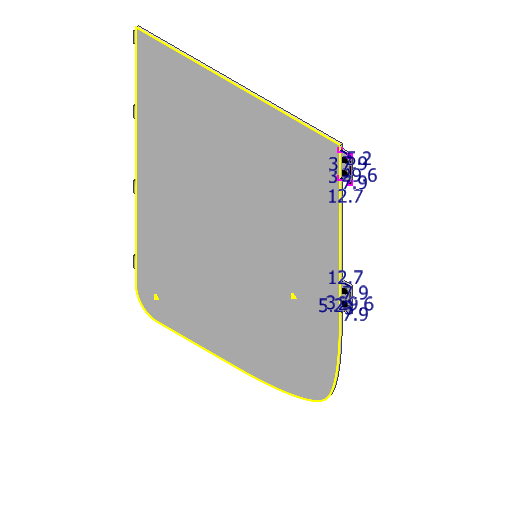
# Autodesk Inventor part: plate cover 1
Saved by Autodesk Inventor 2025.3 (Build 293356030, 356C)
## iProperties
Created: 2025-10-11
Part Number: plate cover 1
Material: 일반
Document SubType Name: Modeling
Designer: joseph
Density: 1 g/cm^3
Appearance: 기본값
Author: joseph
Autodesk Inventor part; units mm, degrees
ref_plane "YZ Plane" through (0, 0, 0) normal (1, 0, 0) x (0, 1, 0)
ref_plane "XZ Plane" through (0, 0, 0) normal (0, 1, 0) x (-1, 0, 0)
ref_plane "XY Plane" through (0, 0, 0) normal (0, 0, 1) x (1, 0, 0)
sketch "스케치1" plane through (0, 0, 0) normal (0, 0, 1) x (1, 0, 0)
  line L0 (-169.6707, -111.8499) -> (-86.0054, -111.8499)
  line L1 (56.3293, 190.1501) -> (-195.6707, 190.1501)
  line L2 (-195.6707, 190.1501) -> (-195.6707, -85.8499)
  arc A0 (-195.6707, -85.8499) -> (-169.6707, -111.8499) centre (-169.6707, -85.8499) ccw
  spline S0 degree 4 poles (76.3293, 10.1501) (76.3293, -29.0333) (69.7342, -103.4516) (54.303, -121.2052) (-24.0976, -131.8499) (-69.6707, -131.8499) knots -3 -3 -3 -3 -3 -2 -1 -1 -1 -1 -1
  line L3 (-169.6707, -111.8499) -> (-69.6707, -111.8499)
  line L4 (56.3293, 10.1501) -> (56.3293, 190.1501)
  line L5 (56.3293, 190.1501) -> (-195.6707, 190.1501)
  line L6 (-195.6707, 190.1501) -> (-195.6707, -85.8499)
  arc A1 (-195.6707, -85.8499) -> (-169.6707, -111.8499) centre (-169.6707, -85.8499) ccw
  spline S1 degree 5 poles (-69.6707, -111.8499) (-63.0133, -111.8499) (-56.3558, -111.7392) (-49.7008, -111.5181) (-37.3206, -110.8938) (-24.9713, -109.8245) (-19.2653, -109.2246) (-9.0381, -107.9323) (1.1128, -106.1432) (5.592, -105.2331) (13.2368, -103.427) (20.711, -101.0169) (23.7891, -99.8797) (28.8563, -97.6943) (33.564, -94.8357) (35.3879, -93.5515) (38.7394, -90.6828) (41.4796, -87.2264) (42.6651, -85.3968) (45.2382, -80.7487) (47.1463, -75.7797) (48.1134, -72.7952) (50.1128, -65.6301) (51.5537, -58.3306) (52.2613, -54.0887) (53.6092, -44.6153) (54.5463, -35.0917) (54.9693, -29.8398) (55.6982, -18.6976) (56.1131, -7.5392) (56.257, -1.6436) (56.3293, 4.2533) (56.3293, 10.1501) knots 0 0 0 0 0 0 0.153999 0.153999 0.153999 0.286688 0.286688 0.286688 0.392369 0.392369 0.392369 0.46822 0.46822 0.46822 0.519585 0.519585 0.519585 0.569776 0.569776 0.569776 0.642294 0.642294 0.642294 0.741735 0.741735 0.741735 0.863596 0.863596 0.863596 1 1 1 1 1 1
  point P0 (-69.6707, -75.8499)
  constraints: 14 end point, 4 point on circle, 2 centre point, 6 other
extrude "돌출1" add sketch "스케치1" along normal blind 3
sketch "스케치2" plane through (-195.6707, -85.8499, 0) normal (-1, 0, 0) x (0, 0, 1)
  line L0 (0, 276) -> (0, 0) projected
  line L1 (0, 0) -> (3, 0) projected
  line L2 (3, 276) -> (3, 0) projected
  line L3 (0, 276) -> (3, 276) projected
  line L4 (0, 276) -> (0, 0) projected
  line L5 (0, 268) -> (-3, 268)
  line L6 (-3, 268) -> (-3, 254)
  line L7 (-3, 254) -> (0, 254)
  line L8 (0, 254) -> (0, 268)
  line L9 (0, 188) -> (-3, 188)
  line L10 (-3, 188) -> (-3, 174)
  line L11 (-3, 174) -> (0, 174)
  line L12 (0, 174) -> (0, 188)
  line L13 (0, 108) -> (-3, 108)
  line L14 (-3, 108) -> (-3, 94)
  line L15 (-3, 94) -> (0, 94)
  line L16 (0, 94) -> (0, 108)
  line L17 (0, 28) -> (-3, 28)
  line L18 (-3, 28) -> (-3, 14)
  line L19 (-3, 14) -> (0, 14)
  line L20 (0, 14) -> (0, 28)
  point P0 (0, 85.8499)
  point P1 (0, 254)
  point P2 (0, 174)
  point P3 (0, 94)
  point P4 (0, 14)
  point P5 (0, 28)
  dimension "d4" = 3
  dimension "d5" = 14
  dimension "d6" = 8
  dimension "d9" = 80
  constraints: 32 end point, 2 parallel, 1 horizontal, 1 perpendicular, 1 point on line, 1 vertical, 24 other
  measures "d4" distance of L7.end L6.end
  measures "d5" distance of L6.end L5.end
  measures "d6" vertical distance of L5.end L0.start
  measures "d9" distance of L5.start L9.start
extrude "돌출2" add sketch "스케치2" against normal blind 20 contours L0 L7 L6 L5 | L0 L11 L10 L9 | L19 L18 L17 L0 | L0 L15 L14 L13
fillet "모깎기1" radius 2 12 edges at (-185.6707, -57.8499, 0) (-175.6707, -64.8499, 0) (-185.6707, -71.8499, 0) (-185.6707, 8.1501, 0) (-175.6707, 15.1501, 0) (-185.6707, 22.1501, 0) (-185.6707, 88.1501, 0) (-175.6707, 95.1501, 0) (-185.6707, 102.1501, 0) (-185.6707, 182.1501, 0) (-175.6707, 175.1501, 0) (-185.6707, 168.1501, 0)
sketch "스케치3" plane through (-195.6707, -85.8499, 3) normal (-1, 0, 0) x (0, 0, 1)
  line L0 (-3, 276) -> (-3, 270) projected
  arc A0 (-5, 268) -> (-3, 270) centre (-5, 270) ccw projected
  line L1 (-5, 268) -> (-6, 268) projected
  line L2 (-6, 268) -> (-6, 254) projected
  line L3 (-6, 254) -> (-5, 254) projected
  arc A1 (-3, 252) -> (-5, 254) centre (-5, 252) ccw projected
  line L4 (-3, 252) -> (-3, 190) projected
  arc A2 (-5, 188) -> (-3, 190) centre (-5, 190) ccw projected
  line L5 (-5, 188) -> (-6, 188) projected
  line L6 (-6, 188) -> (-6, 174) projected
  line L7 (-6, 174) -> (-5, 174) projected
  arc A3 (-3, 172) -> (-5, 174) centre (-5, 172) ccw projected
  line L8 (-3, 172) -> (-3, 110) projected
  arc A4 (-5, 108) -> (-3, 110) centre (-5, 110) ccw projected
  line L9 (-5, 108) -> (-6, 108) projected
  line L10 (-6, 108) -> (-6, 94) projected
  line L11 (-6, 94) -> (-5, 94) projected
  arc A5 (-3, 92) -> (-5, 94) centre (-5, 92) ccw projected
  line L12 (-3, 92) -> (-3, 30) projected
  arc A6 (-5, 28) -> (-3, 30) centre (-5, 30) ccw projected
  line L13 (-5, 28) -> (-6, 28) projected
  line L14 (-6, 28) -> (-6, 14) projected
  line L15 (-6, 14) -> (-5, 14) projected
  arc A7 (-3, 12) -> (-5, 14) centre (-5, 12) ccw projected
  line L16 (-3, 12) -> (-3, 0) projected
  line L17 (-3, 0) -> (0, 0) projected
  line L18 (0, 276) -> (0, 0) projected
  line L19 (-3, 276) -> (0, 276) projected
  line L20 (-6, 14.15) -> (-3.2, 14.15)
  line L21 (-3.2, 14.15) -> (-3.2, 27.85)
  line L22 (-3.2, 27.85) -> (-6, 27.85)
  line L23 (-6, 27.85) -> (-6, 14.15)
  line L24 (-3.2, 107.85) -> (-6, 107.85)
  line L25 (-6, 94.15) -> (-3.2, 94.15)
  line L26 (-6, 107.85) -> (-6, 94.15)
  line L27 (-3.2, 94.15) -> (-3.2, 107.85)
  line L28 (-3.2, 187.85) -> (-6, 187.85)
  line L29 (-6, 174.15) -> (-3.2, 174.15)
  line L30 (-6, 187.85) -> (-6, 174.15)
  line L31 (-3.2, 174.15) -> (-3.2, 187.85)
  line L32 (-3.2, 267.85) -> (-6, 267.85)
  line L33 (-6, 254.15) -> (-3.2, 254.15)
  line L34 (-6, 267.85) -> (-6, 254.15)
  line L35 (-3.2, 254.15) -> (-3.2, 267.85)
  point P0 (-3, 85.8499)
  point P1 (-6, 21)
  point P2 (-6, 101)
  point P3 (-6, 181)
  point P4 (-6, 261)
  point P5 (-6, 267.85)
  point P6 (-6, 27.85)
  dimension "d17" = 2.8
  dimension "d18" = 13.7
  dimension "d21" = 80
  constraints: 32 end point, 2 midpoint, 2 parallel, 1 horizontal, 1 perpendicular, 1 point on line, 1 vertical, 27 other
  measures "d17" distance of L22.end L21.end
  measures "d18" distance of L21.end L20.end
  measures "d21" distance of L22.end L24.end
extrude "돌출3" add sketch "스케치3" along normal blind 6 contours L32 L35 L33 L2 | L14 L22 L21 L20 | L28 L31 L29 L6 | L10 L24 L27 L25
fillet "모깎기3" radius 2 4 edges at (-201.6707, 175.1501, -3) (-201.6707, 95.1501, -3) (-201.6707, 15.1501, -3) (-201.6707, -64.8499, -3)
sketch "스케치5" plane through (0, 0, 3) normal (0, 0, 1) x (1, 0, 0)
  line L0 (56.3293, 190.1501) -> (-195.6707, 190.1501) projected
  line L1 (-195.6707, 190.1501) -> (-195.6707, -85.8499) projected
  arc A0 (-195.6707, -85.8499) -> (-169.6707, -111.8499) centre (-169.6707, -85.8499) ccw projected
  line L2 (-169.6707, -111.8499) -> (-69.6707, -111.8499) projected
  line L3 (56.3293, 10.1501) -> (56.3293, 190.1501) projected
  line L4 (56.4293, 184.9501) -> (69.1293, 184.9501)
  line L5 (69.1293, 184.9501) -> (69.1293, 155.3501)
  line L6 (69.1293, 155.3501) -> (56.4293, 155.3501)
  line L7 (56.3293, 15.3501) -> (69.0293, 15.3501)
  line L8 (69.0293, 15.3501) -> (69.0293, 44.9501)
  line L9 (69.0293, 44.9501) -> (56.3293, 44.9501)
  line L10 (56.3293, 44.9501) -> (56.3293, 15.3501)
  line L11 (56.4293, 184.9501) -> (56.3293, 184.9501)
  line L12 (56.4293, 155.3501) -> (56.3293, 155.3501)
  point P0 (0, 0)
  dimension "d30" = 12.7
  dimension "d31" = 29.6
  dimension "d32" = 5.2
  dimension "d33" = 12.7
  dimension "d34" = 29.6
  dimension "d35" = 5.2
  constraints: 18 end point, 4 perpendicular, 3 parallel, 3 point on line, 2 horizontal, 1 other
  measures "d30" distance of L5.end L6.end
  measures "d31" distance of L4.end L5.end
  measures "d32" distance from line of L0.start L4
  measures "d33" distance of L9.end L8.end
  measures "d34" distance of L8.end L7.end
  measures "d35" distance from line of L3.start L7
extrude "돌출4" add sketch "스케치5" against normal blind 3 contours L3 L9 L8 L7
sketch "스케치6" plane through (0, 0, 3) normal (0, 0, 1) x (1, 0, 0)
  line L0 (56.4293, 155.3501) -> (69.1293, 155.3501) projected
  line L1 (69.1293, 155.3501) -> (69.1293, 184.9501) projected
  line L2 (69.1293, 184.9501) -> (56.4293, 184.9501) projected
  line L3 (56.4293, 184.9501) -> (56.4293, 155.3501) projected
  line L4 (56.3293, 190.1501) -> (-195.6707, 190.1501) projected
  line L5 (-195.6707, 190.1501) -> (-195.6707, -85.8499) projected
  arc A0 (-195.6707, -85.8499) -> (-169.6707, -111.8499) centre (-169.6707, -85.8499) ccw projected
  line L6 (-169.6707, -111.8499) -> (-69.6707, -111.8499) projected
  line L7 (56.3293, 10.1501) -> (56.3293, 15.3501) projected
  line L8 (56.3293, 15.3501) -> (69.0293, 15.3501) projected
  line L9 (69.0293, 15.3501) -> (69.0293, 44.9501) projected
  line L10 (69.0293, 44.9501) -> (56.3293, 44.9501) projected
  line L11 (56.3293, 44.9501) -> (56.3293, 190.1501) projected
  circle A1 centre (62.6793, 177.0501) radius 1.5
  circle A2 centre (62.6793, 163.2501) radius 1.5
  circle A3 centre (62.6793, 37.0501) radius 1.5
  circle A4 centre (62.6793, 23.2501) radius 1.5
  point P0 (0, 0)
  dimension "d38" = 3
  dimension "d39" = 3
  dimension "d40" = 7.9
  dimension "d41" = 7.9
  dimension "d42" = 3
  dimension "d43" = 3
  dimension "d44" = 7.9
  dimension "d45" = 7.9
  constraints: 4 centre point, 1 other
  measures "d38" diameter of A1
  measures "d39" diameter of A2
  measures "d40" vertical distance of L1.end A1.centre
  measures "d41" distance from line of L0 A2.centre
  measures "d42" diameter of A3
  measures "d43" diameter of A4
  measures "d44" vertical distance of L9.end A3.centre
  measures "d45" vertical distance of L8.end A4.centre
extrude "돌출5" cut sketch "스케치6" against normal through all contours L3 L2 L1 L0 | A1 | A2 | A3 | A4
fillet "모깎기4" radius 2 2 edges at (61.1793, 37.0501, 3) (61.1793, 23.2501, 3) inverted yes
extrude "돌출6" add sketch "스케치5" against normal blind 3 contours L3 L11 L4 L5 L6 L12
extrude "돌출7" cut sketch "스케치6" against normal through all contours A1 | A2
fillet "모깎기5" radius 2 2 edges at (61.1793, 163.2501, 3) (61.1793, 177.0501, 3) inverted yes
